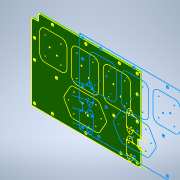
# Autodesk Inventor part: ICU_PDU_PCB
Saved by Autodesk Inventor 2021 (Build 250183000, 183)
## iProperties
Created: 2020-02-27
Part Number: ICU_PDU_PCB
Material: Generic
Document SubType Name: Modeling
Designer: lgnds
Density: 1 g/cm^3
Appearance: Default
Author: lgnds
Autodesk Inventor part; units mm, degrees
ref_plane "YZ Plane" through (0, 0, 0) normal (1, 0, 0) x (0, 1, 0)
ref_plane "XZ Plane" through (0, 0, 0) normal (0, 1, 0) x (-1, 0, 0)
ref_plane "XY Plane" through (0, 0, 0) normal (0, 0, 1) x (1, 0, 0)
sketch "Sketch1" plane through (0, 0, 0) normal (0, 0, 1) x (1, 0, 0)
  line L0 (-69, -79.6965) -> (69, -79.6965)
  line L1 (69, -79.6965) -> (69, 79.6965)
  line L2 (69, 79.6965) -> (-69, 79.6965)
  line L3 (-69, 79.6965) -> (-69, -79.6965)
  line L4 (-69, -79.6965) -> (69, 79.6965) construction
  line L5 (69, -79.6965) -> (-69, 79.6965) construction
  point P0 (0, 0)
  dimension "d0" = 138
  dimension "d1" = 159.393
  constraints: 12 end point, 2 midpoint, 2 parallel, 1 horizontal, 1 perpendicular
  measures "d0" distance of L1.end L2.end
  measures "d1" distance of L2.end L0.start
extrude "Extrusion1" add sketch "Sketch1" along normal blind 1.6
sketch "Sketch2" plane through (0, 0, 1.6) normal (0, 0, 1) x (1, 0, 0)
  line L0 (-69, -79.6965) -> (69, -79.6965) projected
  line L1 (69, -79.6965) -> (-23, -79.6965)
  line L2 (-23, -79.6965) -> (-23, -26.0895)
  line L3 (-23, -26.0895) -> (69, -26.0895)
  line L4 (69, -26.0895) -> (69, -79.6965)
  point P0 (0, 0)
  dimension "d4" = 53.607
  dimension "d5" = 92
  constraints: 8 end point, 2 parallel, 1 horizontal, 1 perpendicular
  measures "d4" distance between parallel lines of L3 L0
  measures "d5" distance of L2.end L3.end
extrude "Extrusion2" cut sketch "Sketch2" against normal blind 1.6
sketch "Sketch3" plane through (0, 0, 1.6) normal (0, 0, 1) x (1, 0, 0)
  line L0 (-86.2964, 75.1965) -> (76.951, 75.1965) construction
  line L1 (69, 79.6965) -> (-69, 79.6965) projected
  circle A0 centre (-42, 75.1965) radius 1.6
  circle A1 centre (42, 75.1965) radius 1.6
  line L2 (-69, 79.6965) -> (-69, -79.6965) projected
  line L3 (69, -26.0895) -> (69, 79.6965) projected
  point P0 (0, 0)
  dimension "d8" = 4.5
  dimension "d9" = 27
  dimension "d10" = 27
  dimension "d11" = 3.2
  dimension "d12" = 3.2
  constraints: 2 centre point, 2 end point, 2 point on line, 1 horizontal
  measures "d8" distance between parallel lines of L1 L0
  measures "d9" distance from line of L2 A0.centre
  measures "d10" distance from line of L3 A1.centre
  measures "d11" diameter of A0
  measures "d12" diameter of A1
extrude "Extrusion3" cut sketch "Sketch3" against normal blind 1.6
sketch "Sketch4" plane through (0, 0, 1.6) normal (0, 0, 1) x (1, 0, 0)
  circle A0 centre (-64.5, 15.6965) radius 2 construction
  circle A1 centre (-64.5, 59.6965) radius 2 construction
  circle A2 centre (0, 75.1965) radius 1.5 construction
  circle A3 centre (64.5, 52.6965) radius 1.5 construction
  circle A4 centre (64.5, 23) radius 1.5 construction
  circle A5 centre (64.5, -21.5906) radius 1.5 construction
  circle A6 centre (42, -21.1966) radius 1.5 construction
  circle A7 centre (-42, -21.5906) radius 1.5 construction
  circle A8 centre (-32, -30.5906) radius 1.5 construction
  circle A9 centre (-32, -75.1966) radius 1.5 construction
  circle A10 centre (-64.5, -52.6966) radius 1.5 construction
  circle A11 centre (-64.5, -30.5906) radius 1.5 construction
  circle A12 centre (-64.5, 25.6965) radius 1.5 construction
  circle A13 centre (-64.5, 49.6965) radius 1.5 construction
  circle A14 centre (-48.8035, -60) radius 7.75 construction
  arc A15 (-64.5, 54.6965) -> (-64.5, 64.6965) centre (-64.5, 59.6965) ccw
  line L0 (-64.5, 64.6965) -> (-69, 64.6965)
  line L1 (-64.5, 54.6965) -> (-69, 54.6965)
  line L2 (-69, 54.6965) -> (-69, 64.6965)
  line L3 (-69, 79.6965) -> (-69, -79.6965) projected
  line L4 (-105.8157, 37.6965) -> (-26.8283, 37.6965) construction
  circle A16 centre (-64.5, 49.6965) radius 1.6
  circle A17 centre (0, 75.1965) radius 1.6
  circle A18 centre (64.5, 52.6965) radius 1.6
  circle A19 centre (-64.5, 15.6965) radius 2 construction
  arc A20 (-64.5, 10.6965) -> (-64.5, 20.6965) centre (-64.5, 15.6965) ccw
  line L5 (-64.5, 10.6965) -> (-69, 10.6965)
  line L6 (-64.5, 20.6965) -> (-69, 20.6965)
  line L7 (-69, 20.6965) -> (-69, 10.6965)
  circle A21 centre (64.5, 23) radius 1.6
  circle A22 centre (64.5, -21.5906) radius 1.6
  circle A23 centre (42, -21.1966) radius 1.6
  circle A24 centre (-42, -21.5906) radius 1.6
  circle A25 centre (-32, -30.5906) radius 1.6
  circle A26 centre (-64.5, -30.5906) radius 1.6
  circle A27 centre (-64.5, -52.6966) radius 1.6
  circle A28 centre (-32, -75.1966) radius 1.5
  circle A29 centre (-48.8035, -60) radius 10
  circle A30 centre (-64.5, 25.6965) radius 1.6
  point P0 (0, 0)
  point P1 (-69, 59.6965)
  point P2 (-69, 15.6965)
  point P3 (-69, -4.3035)
  dimension "d15" = 10
  dimension "d16" = 22
  dimension "d17" = 44
  dimension "d18" = 3.2
  dimension "d19" = 3.2
  dimension "d20" = 3.2
  dimension "d21" = 3.2
  dimension "d22" = 3.2
  dimension "d23" = 3.2
  dimension "d24" = 3.2
  dimension "d25" = 3.2
  dimension "d26" = 3.2
  dimension "d27" = 3.2
  dimension "d28" = 20
  dimension "d29" = 3.2
  constraints: 16 centre point, 15 coincident, 14 end point, 8 symmetric about line, 4 point on circle, 3 horizontal, 2 tangent, 1 concentric, 1 midpoint, 1 point on line, 1 vertical, 2 other
  measures "d15" diameter of A15
  measures "d16" distance from line of L4 A1.centre
  measures "d17" distance of A1.centre A0.centre
  measures "d18" diameter of A16
  measures "d19" diameter of A17
  measures "d20" diameter of A18
  measures "d21" diameter of A26
  measures "d22" diameter of A25
  measures "d23" diameter of A24
  measures "d24" diameter of A23
  measures "d25" diameter of A22
  measures "d26" diameter of A21
  measures "d27" diameter of A27
  measures "d28" diameter of A29
  measures "d29" diameter of A30
extrude "Extrusion4" cut sketch "Sketch4" against normal up to next
sketch "Sketch5" plane through (0, 0, 1.6) normal (0, 0, 1) x (1, 0, 0)
  line L0 (-69, -79.6965) -> (-23, -79.6965) projected
  line L1 (-23, -26.0895) -> (-27.5, -26.0895)
  line L2 (-27.5, -26.0895) -> (-27.5, -79.6965)
  line L3 (-27.5, -79.6965) -> (-23, -79.6965)
  line L4 (-23, -79.6965) -> (-23, -26.0895)
  circle A0 centre (-32, -30.5906) radius 1.6 projected
  point P0 (0, 0)
  dimension "d32" = 4.5
  constraints: 8 end point, 2 parallel, 1 horizontal, 1 perpendicular, 1 point on line
  measures "d32" distance from line of L2 A0.centre
extrude "Extrusion5" cut sketch "Sketch5" against normal up to next contours L2 L1 L4 L0
thicken "Thicken1" operation add thickness 0.75 both sides no extend neighbours yes toward (0, 1, 0) faces at (-55.1667, -79.6965, 0.5333) (-69, -19.4345, 1.0667) (-27.5, -43.9585, 1.0667) (4.6667, -26.0895, 1.0667) (69, 9.1725, 0.5333) (23, 79.6965, 1.0667) (-69, 74.6965, 0.5333)
thicken "Thicken2" operation add thickness 0.75 both sides no extend neighbours yes toward (1, 0, 0) faces at (-69, 43.3632, 1.0667)
sketch "Sketch6" plane through (0, 0, 1.6) normal (0, 0, 1) x (1, 0, 0)
  line L0 (-68.25, 10.6965) -> (-68.25, -78.9465) construction
  line L1 (-28.25, -25.3395) -> (-68.25, -25.3395)
  line L2 (-28.25, -78.9465) -> (-28.25, -25.3395) projected
  line L3 (-68.25, -78.9465) -> (-28.25, -78.9465) projected
  line L4 (-68.25, -25.3395) -> (-68.25, -78.9465)
  point P0 (0, 0)
  constraints: 4 end point, 1 horizontal, 1 point on line, 1 vertical
extrude "Extrusion6" cut sketch "Sketch6" against normal blind 10
sketch "Sketch7" plane through (0, 0, 1.6) normal (0, 0, 1) x (1, 0, 0)
  circle A0 centre (-42, -21.5906) radius 1.6
  line L0 (-68.25, 10.6965) -> (-68.25, 64.6965) projected
  line L1 (-28.25, -25.3395) -> (68.25, -25.3395) projected
  circle A1 centre (-42, -21.5906) radius 1.6 projected
  circle A2 centre (0, 75.1965) radius 1.6 projected
  point P0 (0, 0)
  point P1 (-68.25, -25.3395)
  dimension "d41" = 3.2
  dimension "d42" = 26.25
  dimension "d43" = 3.7489
  dimension "d44" = 3.7489
  dimension "d83" = 3.2
  constraints: 1 centre point
  measures "d41" diameter of A0
  measures "d42" distance from line of L0 A0.centre
  measures "d43" distance from line of L1 A0.centre
  measures "d44" distance from line of L1 A1.centre
  measures "d83" diameter of A2
extrude "Extrusion7" cut sketch "Sketch7" against normal blind 10 contours A0
sketch "Sketch8" plane through (0, 0, 1.6) normal (0, 0, 1) x (1, 0, 0)
  line L0 (-28.25, -25.3395) -> (68.25, -25.3395) projected
  line L1 (55.25, -25.3395) -> (55.25, 39.5162)
  line L2 (68.25, -11) -> (43.3361, -11)
  line L3 (68.25, 18.696) -> (45.1174, 18.696)
  line L4 (68.25, -25.3395) -> (68.25, 78.9465) projected
  point P0 (0, 0)
  point P1 (-68.25, -25.3395)
  dimension "d51" = 55.25
  dimension "d52" = 11
  dimension "d53" = 29.696
  constraints: 6 end point, 2 horizontal, 1 point on line, 1 vertical
  measures "d51" distance from line of point (0, 0) L1
  measures "d52" distance from line of point (0, 0) L2
  measures "d53" distance between parallel lines of L2 L3
fillet "Fillet1" radius 1 6 edges at (68.25, -25.3395, 0.8) (68.25, 78.9465, 0.8) (-68.25, 64.6965, 0.8) (-68.25, 54.6965, 0.8) (-68.25, 20.6965, 0.8) (-68.25, 10.6965, 0.8)
sketch "Sketch9" plane through (0, 0, 1.6) normal (0, 0, 1) x (1, 0, 0)
  line L0 (-68.25, 78.9465) -> (-59.25, 78.9465)
  line L1 (-59.25, 78.9465) -> (-59.25, 69.9465)
  line L2 (-59.25, 69.9465) -> (-68.25, 69.9465)
  line L3 (-68.25, 69.9465) -> (-68.25, 78.9465)
  line L4 (68.25, -24.3395) -> (68.25, 77.9465) projected
  line L5 (68.25, -24.3395) -> (68.25, 77.9465) projected
  line L6 (64.5, -4.5535) -> (68.25, -4.5535)
  line L7 (68.25, -4.5535) -> (68.25, 4.4465)
  line L8 (68.25, 4.4465) -> (64.5, 4.4465)
  line L9 (64.5, 4.4465) -> (64.5, -4.5535)
  line L10 (64.5, -4.5535) -> (68.25, 4.4465) construction
  line L11 (68.25, -4.5535) -> (64.5, 4.4465) construction
  line L12 (67.25, 78.9465) -> (-68.25, 78.9465) projected
  point P0 (0, 0)
  point P1 (66.375, -0.0535)
  dimension "d57" = 9
  dimension "d58" = 9
  dimension "d74" = 9
  dimension "d75" = 3.75
  dimension "d76" = 79
  constraints: 20 end point, 4 parallel, 2 horizontal, 2 midpoint, 2 perpendicular, 1 point on line
  measures "d57" distance of L0.end L1.end
  measures "d58" distance of L1.end L2.end
  measures "d74" distance of L8.end L6.start
  measures "d75" distance of L7.end L8.end
  measures "d76" distance from line of L12 point (66.375, -0.053)
extrude "Extrusion8" cut sketch "Sketch9" against normal blind 10
fillet "Fillet3" radius 1 3 edges at (-68.25, 69.9465, 0.8) (-59.25, 78.9465, 0.8) (-59.25, 69.9465, 0.8)
sketch "Sketch10" plane through (0, 0, 1.6) normal (0, 0, 1) x (1, 0, 0)
  circle A0 centre (-42, -21.5906) radius 1.6 construction
  circle A1 centre (-64.5, 25.6965) radius 1.6 construction
  line L0 (-64.5, 25.6965) -> (-64.5, -21.5906) construction
  line L1 (-64.5, -21.5906) -> (-42, -21.5906) construction
  circle A2 centre (42, 75.1965) radius 1.6 construction
  circle A3 centre (64.5, 52.6965) radius 1.6 construction
  line L2 (42, 75.1965) -> (64.5, 75.1965) construction
  line L3 (64.5, 75.1965) -> (64.5, 52.6965) construction
  circle A4 centre (-64.5, -21.5906) radius 1.6
  circle A5 centre (64.5, 75.1965) radius 1.6
  point P0 (0, 0)
  dimension "d62" = 3.2
  dimension "d63" = 3.2
  dimension "d64" = 3.2
  constraints: 8 end point, 2 centre point, 2 coincident, 2 perpendicular, 1 horizontal, 1 vertical
  measures "d62" diameter of A1
  measures "d63" diameter of A4
  measures "d64" diameter of A5
extrude "Extrusion9" cut sketch "Sketch10" against normal up to next
fillet "Fillet6" radius 1 4 edges at (64.5, 4.4465, 0.8) (68.25, 4.4465, 0.8) (64.5, -4.5535, 0.8) (68.25, -4.5535, 0.8)
sketch "Sketch12" plane through (0, 0, 1.6) normal (0, 0, 1) x (1, 0, 0)
  circle A0 centre (-37, 19.9095) radius 1.6
  circle A1 centre (-42, -21.5906) radius 1.6 projected
  circle A2 centre (-64.5, -21.5906) radius 1.6 projected
  line L0 (-68.25, 9.6965) -> (-68.25, 21.6965) projected
  line L1 (67.25, 78.9465) -> (-58.25, 78.9465) projected
  circle A3 centre (35, 14.9095) radius 1.6
  line L2 (-68.25, -25.3395) -> (67.25, -25.3395) projected
  line L3 (68.25, 5.4465) -> (68.25, 77.9465) projected
  point P0 (0, 0)
  point P1 (-68.25, -24.3395)
  point P2 (-67.25, -25.3395)
  dimension "d78" = 3.2
  dimension "d79" = 3.2
  dimension "d80" = 3.2
  dimension "d81" = 31.25
  dimension "d82" = 59.037
  dimension "d84" = 40.249
  dimension "d85" = 33.25
  dimension "d86" = 3.2
  constraints: 2 centre point
  measures "d78" diameter of A0
  measures "d79" diameter of A1
  measures "d80" diameter of A2
  measures "d81" distance from line of L0 A0.centre
  measures "d82" distance from line of L1 A0.centre
  measures "d84" distance from line of L2 A3.centre
  measures "d85" distance from line of L3 A3.centre
  measures "d86" diameter of A3
extrude "Extrusion11" cut sketch "Sketch12" against normal blind 10 contours A0 | A3
sketch "Sketch13" plane through (0, 0, 1.6) normal (0, 0, 1) x (1, 0, 0)
  circle A0 centre (42, -21.1966) radius 1.6 projected
  point P0 (0, 0)
extrude "Extrusion12" add sketch "Sketch13" against normal up to surface (1.6 mm away)
sketch "Sketch14" plane through (0, 0, 1.6) normal (0, 0, 1) x (1, 0, 0)
  circle A0 centre (64.5, -21.5906) radius 1.6 construction
  line L0 (64.5, -21.5906) -> (-20.9214, -21.5906) construction
  circle A1 centre (0, -21.5906) radius 1.6
  circle A2 centre (42, -21.5906) radius 1.6
  point P0 (0, 0)
  dimension "d91" = 3.2
  dimension "d92" = 3.2
  dimension "d93" = 3.2
  dimension "d94" = 22.5
  dimension "d95" = 42
  constraints: 2 centre point, 2 end point, 2 point on line, 1 horizontal
  measures "d91" diameter of A0
  measures "d92" diameter of A2
  measures "d93" diameter of A1
  measures "d94" distance of L0.start A2.centre
  measures "d95" distance of A2.centre A1.centre
extrude "Extrusion13" cut sketch "Sketch14" against normal up to next
sketch "Sketch16" plane through (0, 0, 1.6) normal (0, 0, 1) x (1, 0, 0)
  circle A0 centre (42, -21.5906) radius 1.6 projected
  point P0 (0, 0)
extrude "Extrusion14" add sketch "Sketch16" against normal up to surface (1.6 mm away)
sketch "Sketch17" plane through (0, 0, 1.6) normal (0, 0, 1) x (1, 0, 0)
  circle A0 centre (0, -21.5906) radius 1.5 projected
  circle A1 centre (64.5, -21.5906) radius 1.5 projected
  circle A2 centre (0, -21.5906) radius 1.6 projected
  line L0 (0, -21.5906) -> (64.5, -21.5906) construction
  circle A3 centre (44, -21.5906) radius 1.6
  point P0 (0, 0)
  dimension "d100" = 44
  dimension "d101" = 3.2
  dimension "d102" = 3.2
  constraints: 2 end point, 1 centre point, 1 horizontal, 1 point on line
  measures "d100" distance of A0.centre A3.centre
  measures "d101" diameter of A3
  measures "d102" diameter of A2
extrude "Extrusion15" cut sketch "Sketch17" against normal blind 10 contours A3
sketch "Sketch18" plane through (0, 0, 1.6) normal (0, 0, 1) x (1, 0, 0)
  line L0 (-68.25, 65.6965) -> (-59.5, 65.6965)
  line L1 (-59.5, 65.6965) -> (-59.5, 53.6965)
  line L2 (-59.5, 53.6965) -> (-68.25, 53.6965)
  line L3 (-68.25, 53.6965) -> (-68.25, 65.6965)
  arc A0 (-64.5, 54.6965) -> (-64.5, 64.6965) centre (-64.5, 59.6965) ccw projected
  line L4 (-68.25, 21.6965) -> (-59.5, 21.6965)
  line L5 (-59.5, 21.6965) -> (-59.5, 9.6965)
  line L6 (-59.5, 9.6965) -> (-68.25, 9.6965)
  line L7 (-68.25, 9.6965) -> (-68.25, 21.6965)
  arc A1 (-64.5, 10.6965) -> (-64.5, 20.6965) centre (-64.5, 15.6965) ccw projected
  point P0 (0, 0)
  constraints: 16 end point, 4 parallel, 2 coincident, 2 horizontal, 2 perpendicular, 2 tangent
extrude "Extrusion16" add sketch "Sketch18" against normal up to surface (1.6 mm away)
sketch "OUTLINE_EXTRA" plane through (0, 0, 1.6) normal (0, 0, 1) x (1, 0, 0)
  circle A0 centre (0, -21.5906) radius 1.6 projected
  circle A1 centre (-37, 19.9095) radius 1.6 projected
  circle A2 centre (35, 14.9095) radius 1.6 projected
  circle A3 centre (42, 75.1965) radius 1.6 projected
  circle A4 centre (-42, 75.1965) radius 1.6 projected
  circle A5 centre (64.5, 23) radius 1.6 projected
  circle A6 centre (0, 75.1965) radius 1.6 projected
  circle A7 centre (-64.5, 49.6965) radius 1.6 projected
  circle A8 centre (64.5, 52.6965) radius 1.6 projected
  circle A9 centre (64.5, -21.5906) radius 1.6 projected
  circle A10 centre (-42, -21.5906) radius 1.6 projected
  circle A11 centre (-64.5, 25.6965) radius 1.6 projected
  circle A12 centre (64.5, 75.1965) radius 1.6 projected
  circle A13 centre (-64.5, -21.5906) radius 1.6 projected
  arc A14 (68.25, -5.5535) -> (67.25, -4.5535) centre (67.25, -5.5535) ccw projected
  line L0 (67.25, -4.5535) -> (65.5, -4.5535) projected
  arc A15 (64.5, -3.5535) -> (65.5, -4.5535) centre (65.5, -3.5535) ccw projected
  line L1 (64.5, -3.5535) -> (64.5, 3.4465) projected
  arc A16 (65.5, 4.4465) -> (64.5, 3.4465) centre (65.5, 3.4465) ccw projected
  line L2 (65.5, 4.4465) -> (67.25, 4.4465) projected
  arc A17 (67.25, 4.4465) -> (68.25, 5.4465) centre (67.25, 5.4465) ccw projected
  line L3 (68.25, 5.4465) -> (68.25, 77.9465) projected
  arc A18 (68.25, 77.9465) -> (67.25, 78.9465) centre (67.25, 77.9465) ccw projected
  line L4 (67.25, 78.9465) -> (-58.25, 78.9465) projected
  arc A19 (-58.25, 78.9465) -> (-59.25, 77.9465) centre (-58.25, 77.9465) ccw projected
  line L5 (-59.25, 77.9465) -> (-59.25, 70.9465) projected
  arc A20 (-60.25, 69.9465) -> (-59.25, 70.9465) centre (-60.25, 70.9465) ccw projected
  line L6 (-60.25, 69.9465) -> (-67.25, 69.9465) projected
  arc A21 (-67.25, 69.9465) -> (-68.25, 68.9465) centre (-67.25, 68.9465) ccw projected
  line L7 (-68.25, 68.9465) -> (-68.25, -25.3395) projected
  line L8 (-68.25, -25.3395) -> (67.25, -25.3395) projected
  arc A22 (67.25, -25.3395) -> (68.25, -24.3395) centre (67.25, -24.3395) ccw projected
  line L9 (68.25, -24.3395) -> (68.25, -5.5535) projected
  line L10 (60.7235, -19.25) -> (77.2235, -23.098) projected
  line L11 (51.7235, -19.25) -> (60.7235, -19.25) projected
  line L12 (51.7235, -19.25) -> (60.7235, -19.25) projected
  line L13 (51.7235, -19.25) -> (60.7235, -19.25) projected
  arc A23 (50.7235, -18.25) -> (51.7235, -19.25) centre (51.7235, -18.25) ccw projected
  line L14 (50.7235, -3.75) -> (50.7235, -18.25) projected
  arc A24 (51.7235, -2.75) -> (50.7235, -3.75) centre (51.7235, -3.75) ccw projected
  line L15 (60.7235, -2.75) -> (51.7235, -2.75) projected
  line L16 (77.2235, -6.598) -> (60.7235, -2.75) projected
  line L17 (60.7235, 10.446) -> (77.2235, 6.598) projected
  line L18 (60.7235, 10.446) -> (77.2235, 6.598) projected
  line L19 (51.7235, 10.446) -> (60.7235, 10.446) projected
  line L20 (51.7235, 10.446) -> (60.7235, 10.446) projected
  arc A25 (50.7235, 11.446) -> (51.7235, 10.446) centre (51.7235, 11.446) ccw projected
  line L21 (50.7235, 25.946) -> (50.7235, 11.446) projected
  arc A26 (51.7235, 26.946) -> (50.7235, 25.946) centre (51.7235, 25.946) ccw projected
  line L22 (60.7235, 26.946) -> (51.7235, 26.946) projected
  line L23 (77.2235, 23.098) -> (60.7235, 26.946) projected
  line L24 (51.3351, 27.3889) -> (52.8256, 30.766) projected
  line L25 (51.3351, 27.3889) -> (52.8256, 30.766) projected
  arc A27 (51.3351, 27.3889) -> (51.25, 26.9851) centre (52.25, 26.9851) ccw projected
  line L26 (51.25, 26.9851) -> (51.25, 25.996) projected
  arc A28 (57.6744, 30.766) -> (52.8256, 30.766) centre (55.25, 29.696) ccw projected
  line L27 (57.6744, 30.766) -> (59.1649, 27.3889) projected
  arc A29 (59.25, 26.9851) -> (59.1649, 27.3889) centre (58.25, 26.9851) ccw projected
  line L28 (59.25, 25.996) -> (59.25, 26.9851) projected
  line L29 (52.8256, 6.626) -> (51.3351, 10.0031) projected
  line L30 (52.8256, 6.626) -> (51.3351, 10.0031) projected
  arc A30 (52.8256, 6.626) -> (57.6744, 6.626) centre (55.25, 7.696) ccw projected
  line L31 (59.1649, 10.0031) -> (57.6744, 6.626) projected
  arc A31 (59.1649, 10.0031) -> (59.25, 10.4069) centre (58.25, 10.4069) ccw projected
  line L32 (59.25, 10.4069) -> (59.25, 11.396) projected
  arc A32 (51.25, 10.4069) -> (51.3351, 10.0031) centre (52.25, 10.4069) ccw projected
  line L33 (51.25, 11.396) -> (51.25, 10.4069) projected
  line L34 (59.75, 26.5685) -> (59.75, 25.296) projected
  line L35 (59.75, 10.8235) -> (59.75, 12.096) projected
  line L36 (59.75, -3.1275) -> (59.75, -4.4) projected
  line L37 (59.75, -18.8725) -> (59.75, -17.6) projected
  line L38 (52.8, -23.01) -> (51.3118, -19.4) projected
  line L39 (52.8, -23.01) -> (51.3118, -19.4) projected
  arc A33 (52.8, -23.01) -> (57.7, -23.01) centre (55.25, -22) ccw projected
  line L40 (57.7, -23.01) -> (59.0914, -19.6347) projected
  arc A34 (59.2907, -19.4) -> (59.0914, -19.6347) centre (59.5537, -19.8253) ccw projected
  arc A35 (57.6744, 1.07) -> (52.8256, 1.07) centre (55.25, 0) ccw projected
  arc A36 (57.6744, 1.07) -> (52.8256, 1.07) centre (55.25, 0) ccw projected
  line L41 (57.6744, 1.07) -> (59.1649, -2.3071) projected
  arc A37 (59.25, -2.7109) -> (59.1649, -2.3071) centre (58.25, -2.7109) ccw projected
  line L42 (59.25, -3.7) -> (59.25, -2.7109) projected
  line L43 (51.3351, -2.3071) -> (52.8256, 1.07) projected
  arc A38 (51.3351, -2.3071) -> (51.25, -2.7109) centre (52.25, -2.7109) ccw projected
  line L44 (51.25, -2.7109) -> (51.25, -3.7) projected
  circle A39 centre (53.75, 24.696) radius 0.49 projected
  circle A40 centre (56.75, 12.696) radius 0.49 projected
  circle A41 centre (56.75, -17) radius 0.49 projected
  circle A42 centre (-4.328, 8.7179) radius 0.944 projected
  circle A43 centre (2.378, -1.4421) radius 0.944 projected
  circle A44 centre (-45.5343, 48.7507) radius 0.7836 projected
  circle A45 centre (-36.4157, 44.3057) radius 0.7836 projected
  circle A46 centre (34.4657, 48.7507) radius 0.7836 projected
  circle A47 centre (43.5843, 39.8607) radius 0.7836 projected
  line L45 (-30.9674, 66.7339) -> (-50.9826, 66.7339) projected
  line L46 (-30.9674, 66.7339) -> (-50.9826, 66.7339) projected
  arc A48 (-23.8554, 59.6219) -> (-30.9674, 66.7339) centre (-30.9674, 59.6219) ccw projected
  arc A49 (-50.9826, 66.7339) -> (-58.0946, 59.6219) centre (-50.9826, 59.6219) ccw projected
  line L47 (-50.9826, 66.7339) -> (-30.9674, 66.7339) projected
  line L48 (-50.9826, 66.7339) -> (-30.9674, 66.7339) projected
  arc A50 (-50.9826, 66.7339) -> (-58.0946, 59.6219) centre (-50.9826, 59.6219) ccw projected
  line L49 (-58.0946, 36.5079) -> (-58.0946, 59.6219) projected
  arc A51 (-58.0946, 36.5079) -> (-50.9826, 29.3959) centre (-50.9826, 36.5079) ccw projected
  line L50 (-30.9674, 29.3959) -> (-50.9826, 29.3959) projected
  arc A52 (-30.9674, 29.3959) -> (-23.8554, 36.5079) centre (-30.9674, 36.5079) ccw projected
  line L51 (-23.8554, 59.6219) -> (-23.8554, 36.5079) projected
  arc A53 (-23.8554, 59.6219) -> (-30.9674, 66.7339) centre (-30.9674, 59.6219) ccw projected
  line L52 (29.0174, 66.7339) -> (49.0326, 66.7339) projected
  line L53 (29.0174, 66.7339) -> (49.0326, 66.7339) projected
  arc A54 (29.0174, 66.7339) -> (21.9054, 59.6219) centre (29.0174, 59.6219) ccw projected
  line L54 (21.9054, 32.0629) -> (21.9054, 59.6219) projected
  arc A55 (21.9054, 32.0629) -> (29.0174, 24.9509) centre (29.0174, 32.0629) ccw projected
  line L55 (49.0326, 24.9509) -> (29.0174, 24.9509) projected
  arc A56 (49.0326, 24.9509) -> (56.1446, 32.0629) centre (49.0326, 32.0629) ccw projected
  line L56 (56.1446, 59.6219) -> (56.1446, 32.0629) projected
  arc A57 (56.1446, 59.6219) -> (49.0326, 66.7339) centre (49.0326, 59.6219) ccw projected
  line L57 (-26.7422, 6.5629) -> (-19.8718, 18.4629) projected
  line L58 (-26.7422, 6.5629) -> (-19.8718, 18.4629) projected
  arc A58 (-26.7422, 6.5629) -> (-26.7422, 0.7129) centre (-21.676, 3.6379) ccw projected
  line L59 (-19.8718, -11.1871) -> (-26.7422, 0.7129) projected
  arc A59 (-19.8718, -11.1871) -> (-14.8055, -14.1121) centre (-14.8055, -8.2621) ccw projected
  line L60 (12.8556, -14.1121) -> (-14.8055, -14.1121) projected
  arc A60 (12.8556, -14.1121) -> (17.9218, -11.1871) centre (12.8556, -8.2621) ccw projected
  line L61 (24.7923, 0.7129) -> (17.9218, -11.1871) projected
  arc A61 (24.7923, 0.7129) -> (24.7923, 6.5629) centre (19.726, 3.6379) ccw projected
  line L62 (17.9218, 18.4629) -> (24.7923, 6.5629) projected
  arc A62 (17.9218, 18.4629) -> (12.8556, 21.3879) centre (12.8556, 15.5379) ccw projected
  line L63 (-14.8055, 21.3879) -> (12.8556, 21.3879) projected
  arc A63 (-14.8055, 21.3879) -> (-19.8718, 18.4629) centre (-14.8055, 15.5379) ccw projected
  circle A64 centre (53.75, -5) radius 0.5193 projected
  circle A65 centre (44, -21.5906) radius 1.6 projected
  circle A66 centre (-5.5343, 48.7507) radius 0.7836 projected
  circle A67 centre (3.5843, 39.8607) radius 0.7836 projected
  arc A68 (-10.9826, 66.7339) -> (-18.0946, 59.6219) centre (-10.9826, 59.6219) ccw projected
  arc A69 (-10.9826, 66.7339) -> (-18.0946, 59.6219) centre (-10.9826, 59.6219) ccw projected
  line L64 (-18.0946, 32.0629) -> (-18.0946, 59.6219) projected
  arc A70 (-18.0946, 32.0629) -> (-10.9826, 24.9509) centre (-10.9826, 32.0629) ccw projected
  line L65 (9.0326, 24.9509) -> (-10.9826, 24.9509) projected
  arc A71 (9.0326, 24.9509) -> (16.1446, 32.0629) centre (9.0326, 32.0629) ccw projected
  line L66 (16.1446, 59.6219) -> (16.1446, 32.0629) projected
  arc A72 (16.1446, 59.6219) -> (9.0326, 66.7339) centre (9.0326, 59.6219) ccw projected
  line L67 (-10.9826, 66.7339) -> (9.0326, 66.7339) projected
  point P0 (0, 0)
equation "\"d10\" = d9"
equation "\"d12\" = d11"
equation "\"d16\" = 0.5 * d17"
equation "\"d19\" = d18"
equation "\"d20\" = d18"
equation "\"d21\" = d18"
equation "\"d22\" = d18"
equation "\"d23\" = d18"
equation "\"d24\" = d20"
equation "\"d25\" = d20"
equation "\"d26\" = d20"
equation "\"d27\" = d21"
equation "\"d29\" = d18"
equation "\"d41\" = d83"
equation "\"d43\" = d44"
equation "\"d58\" = d57"
equation "\"d74\" = d57"
equation "\"d63\" = d62"
equation "\"d64\" = d62"
equation "\"d78\" = d80"
equation "\"d86\" = d79"
equation "\"d92\" = d91"
equation "\"d93\" = d91"
equation "\"d101\" = d102"
body "Solid1"
